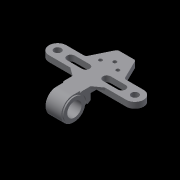
# Autodesk Inventor part: PelvisSpineLink
Saved by Autodesk Inventor 2015 (Build 190159000, 159)
## iProperties
RuleStatus: InUse
Created: 2014-12-14
Part Number: PelvisSpineLink
Material: Generic
Document SubType Name: Modeling
Designer: Inventor
Mass: 10.3501 g
Surface Area: 65.2714 cm^2
Volume: 10.3501 cm^3
Density: 1 g/cm^3
Appearance: Default
BeforeDocSave0: UpdateBoundingBox
CX: 79.00 mm
CY: 61.00 mm
CZ: 20.00 mm
Author: Inventor
Autodesk Inventor part; units mm, degrees
ref_plane "YZ Plane" through (0, 0, 0) normal (1, 0, 0) x (0, 1, 0)
ref_plane "XZ Plane" through (0, 0, 0) normal (0, 1, 0) x (-1, 0, 0)
sketch "Body" plane through (0, 0, 0) normal (0, 0, 1) x (1, 0, 0)
  line L0 (-42.1685, 50.6373) -> (57.8315, 50.6373) construction
  line L1 (-42.1685, 50.6373) -> (-42.1685, 45.6373) construction
  line L2 (-42.1685, 45.6373) -> (-31.6685, 45.6373) construction
  line L3 (-31.6685, 45.6373) -> (-31.6685, 18.1373) construction
  line L4 (-31.6685, 18.1373) -> (-42.1685, 18.1373) construction
  line L5 (-42.1685, 18.1373) -> (-42.1685, 13.1373) construction
  line L6 (-42.1685, 13.1373) -> (57.8315, 13.1373) construction
  line L7 (57.8315, 18.1373) -> (57.8315, 13.1373) construction
  line L8 (47.3315, 18.1373) -> (57.8315, 18.1373) construction
  line L9 (47.3315, 45.6373) -> (47.3315, 18.1373) construction
  line L10 (57.8315, 45.6373) -> (47.3315, 45.6373) construction
  line L11 (57.8315, 50.6373) -> (57.8315, 45.6373) construction
  circle A0 centre (40.0815, 25.3873) radius 3.25 construction
  arc A1 (28.5815, 34.3873) -> (28.5815, 37.8873) centre (28.5815, 36.1373) ccw construction
  line L12 (15.0815, 34.3873) -> (28.5815, 34.3873) construction
  arc A2 (15.0815, 37.8873) -> (15.0815, 34.3873) centre (15.0815, 36.1373) ccw construction
  line L13 (28.5815, 37.8873) -> (15.0815, 37.8873) construction
  line L14 (29.0815, 28.6373) -> (16.5815, 28.6373) projected
  arc A3 (29.0815, 22.1373) -> (29.0815, 28.6373) centre (29.0815, 25.3873) ccw projected
  line L15 (16.5815, 22.1373) -> (29.0815, 22.1373) projected
  arc A4 (16.5815, 28.6373) -> (16.5815, 22.1373) centre (16.5815, 25.3873) ccw projected
  line L16 (-13.4185, 28.6373) -> (-0.9185, 28.6373) projected
  arc A5 (-0.9185, 22.1373) -> (-0.9185, 28.6373) centre (-0.9185, 25.3873) ccw projected
  line L17 (-0.9185, 22.1373) -> (-13.4185, 22.1373) projected
  arc A6 (-13.4185, 28.6373) -> (-13.4185, 22.1373) centre (-13.4185, 25.3873) ccw projected
  arc A7 (-12.9185, 37.8873) -> (-12.9185, 34.3873) centre (-12.9185, 36.1373) ccw construction
  line L18 (-12.9185, 37.8873) -> (0.5815, 37.8873) construction
  arc A8 (0.5815, 34.3873) -> (0.5815, 37.8873) centre (0.5815, 36.1373) ccw construction
  line L19 (0.5815, 34.3873) -> (-12.9185, 34.3873) construction
  circle A9 centre (-24.4185, 25.3873) radius 3.25 construction
  line L20 (6.8315, 42.6373) -> (8.8315, 42.6373) construction
  arc A10 (8.8315, 39.1373) -> (8.8315, 42.6373) centre (8.8315, 40.8873) ccw construction
  line L21 (6.8315, 39.1373) -> (8.8315, 39.1373) construction
  arc A11 (6.8315, 42.6373) -> (6.8315, 39.1373) centre (6.8315, 40.8873) ccw construction
  circle A12 centre (40.0815, 25.3873) radius 7.25
  circle A13 centre (-24.4185, 25.3873) radius 7.25
  line L22 (40.0815, 25.3873) -> (40.0815, 18.1373) construction
  line L23 (-24.4185, 18.1373) -> (40.0815, 18.1373)
  line L24 (-24.4185, 25.3873) -> (-24.4185, 18.1373) construction
  line L25 (40.0815, 25.3873) -> (40.0815, 32.6373) construction
  line L26 (-24.4185, 25.3873) -> (-24.4185, 32.6373) construction
  line L27 (40.0815, 32.6373) -> (24.0815, 32.6373)
  line L28 (24.0815, 32.6373) -> (15.3024, 50.6373)
  line L29 (15.3024, 50.6373) -> (0.3607, 50.6373)
  line L30 (0.3607, 50.6373) -> (-8.4185, 32.6373)
  line L31 (-8.4185, 32.6373) -> (-24.4185, 32.6373)
  line L32 (8.8315, 40.8873) -> (6.8315, 40.8873) construction
  circle A14 centre (7.8315, 40.8873) radius 1.5
  circle A15 centre (0.5815, 36.1373) radius 1.5
  circle A16 centre (15.0815, 36.1373) radius 1.5
  circle A17 centre (40.0815, 25.3873) radius 3
  circle A18 centre (-24.4185, 25.3873) radius 3
  dimension "d2" = 16
  dimension "d3" = 16
  dimension "d4" = 116
  dimension "d8" = 3
  dimension "d9" = 3
  dimension "d10" = 3
  dimension "d11" = 6
  dimension "d12" = 6
  constraints: 22 end point, 7 centre point, 6 coincident, 4 point on circle, 4 tangent, 4 vertical, 2 horizontal, 2 point on line, 1 equal length, 1 midpoint, 1 parallel, 1 perpendicular
  measures "d2" distance of L25.end L27.end
  measures "d3" distance of L30.end L26.end
  measures "d4" angle of L28 L27
  measures "d8" diameter of A14
  measures "d9" diameter of A15
  measures "d10" diameter of A16
  measures "d11" diameter of A17
  measures "d12" diameter of A18
extrude "BodyFeature" add sketch "Body" along normal blind 5
fillet "BodyFilletsFeature" radius 2 4 edges at (24.0815, 32.6373, 2.5) (-8.4185, 32.6373, 2.5) (0.3607, 50.6373, 2.5) (15.3024, 50.6373, 2.5)
ref_plane "MiddlePlane" through (7.8315, 65.9547, 5) normal (1, 0, 0) x (0, 0, -1)
sketch "PelvisSpineBase" plane through (7.8315, 65.9547, 5) normal (1, 0, 0) x (0, 0, -1)
  arc A0 (0, -66.3174) -> (12.5911, -56.659) centre (10, -66.3174) ccw
  circle A1 centre (10, -66.3174) radius 6
  line L0 (5, -33.3174) -> (5, -47.8174) construction
  line L1 (5, -47.8174) -> (0, -47.8174)
  line L2 (0, -47.8174) -> (0, -66.3174)
  line L3 (5, -47.8174) -> (5, -52.8174)
  line L4 (5, -52.8174) -> (10, -52.8174)
  line L5 (10, -52.8174) -> (12.5911, -56.659)
  dimension "d16" = 12
  dimension "d17" = 4
  dimension "d22" = 5
  dimension "d23" = 5
  dimension "d29" = 18.5
  dimension "d30" = 34
  constraints: 10 end point, 2 centre point, 2 horizontal, 2 point on circle, 2 vertical, 1 coincident, 1 tangent
  measures "d16" diameter of A1
  measures "d17" radial gap between concentric circles of A0 A1
  measures "d22" distance of L0.end L3.end
  measures "d23" distance of L3.end L4.end
  measures "d29" distance of L1.end L2.end
  measures "d30" angle of L2 L5
extrude "PelvisSpineBaseFeature" add sketch "PelvisSpineBase" along normal mid plane 15
sketch "AngleReinforce" plane through (0, 0, 5) normal (0, 0, 1) x (1, 0, 0)
  line L0 (15.3315, 18.1373) -> (15.3315, 13.1373)
  line L1 (15.3315, 13.1373) -> (15.3315, 18.1373) projected
  line L2 (15.3315, 13.1373) -> (22.3315, 18.1373)
  line L3 (15.3315, 18.1373) -> (40.0815, 18.1373) construction
  line L4 (15.3315, 18.1373) -> (22.3315, 18.1373)
  line L5 (0.3315, 18.1373) -> (0.3315, 13.1373)
  line L6 (0.3315, 18.1373) -> (0.3315, 13.1373) projected
  line L7 (0.3315, 13.1373) -> (-6.6685, 18.1373)
  line L8 (-24.4185, 18.1373) -> (0.3315, 18.1373) construction
  line L9 (0.3315, 18.1373) -> (-6.6685, 18.1373)
  dimension "d33" = 7
  dimension "d34" = 7
  constraints: 12 end point, 4 collinear, 2 point on line
  measures "d33" horizontal distance of L0.end L2.end
  measures "d34" horizontal distance of L5.end L7.end
extrude "AngleReinforceFeature" add sketch "AngleReinforce" against normal blind 2
sketch "RightLip" plane through (15.3315, 65.9547, 5) normal (1, 0, 0) x (0, 0, -1)
  arc A0 (0, -66.3174) -> (12.5911, -56.659) centre (10, -66.3174) ccw projected
  circle A1 centre (10, -66.3174) radius 10
  circle A2 centre (10, -66.3174) radius 9
  dimension "d37" = 1
  constraints: 2 centre point, 2 coincident, 1 concentric
  measures "d37" radial gap between concentric circles of A0 A2
extrude "RightLipFeature" cut sketch "RightLip" against normal blind 1
sketch "LeftLip" plane through (0.3315, 65.9547, 5) normal (-1, 0, 0) x (0, 0, 1)
  arc A0 (-12.5911, -56.659) -> (0, -66.3174) centre (-10, -66.3174) ccw projected
  circle A1 centre (-10, -66.3174) radius 9
  circle A2 centre (-10, -66.3174) radius 10
  dimension "d40" = 1
  constraints: 2 centre point, 2 coincident, 1 concentric
  measures "d40" radial gap between concentric circles of A0 A1
extrude "LeftLipFeature" cut sketch "LeftLip" against normal blind 1
fillet "SharpEdgesFilletFeature" radius 1 4 edges at (0.8315, -0.3627, 5) (0.8315, 9.2958, -7.5911) (14.8315, 9.2958, -7.5911) (14.8315, -0.3627, 5)
equation "\"d3\" = d2"
